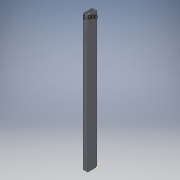
# Autodesk Inventor part: 30in 1x1 Beam
Saved by Autodesk Inventor 2018 (Build 220112000, 112)
## iProperties
Created: 2019-01-16
Part Number: 30in 1x1 Beam
Material: Generic
Document SubType Name: Modeling
Designer: Gabriel
Density: 1 g/cm^3
Appearance: Default
Author: Gabriel
Autodesk Inventor part; units mm, degrees
ref_plane "YZ Plane" through (0, 0, 0) normal (1, 0, 0) x (0, 1, 0)
ref_plane "XZ Plane" through (0, 0, 0) normal (0, 1, 0) x (-1, 0, 0)
ref_plane "XY Plane" through (0, 0, 0) normal (0, 0, 1) x (1, 0, 0)
sketch "Sketch1" plane through (0, 0, 0) normal (0, 1, 0) x (-1, 0, 0)
  line L0 (2.2807, -2.5252) -> (-23.1193, -2.5252)
  line L1 (-23.1193, -2.5252) -> (-23.1193, 48.2748)
  line L2 (-23.1193, 48.2748) -> (2.2807, 48.2748)
  line L3 (2.2807, 48.2748) -> (2.2807, -2.5252)
  line L4 (-19.9443, 0.6498) -> (-0.8943, 0.6498)
  line L5 (-0.8943, 0.6498) -> (-0.8943, 45.0998)
  line L6 (-0.8943, 45.0998) -> (-19.9443, 45.0998)
  line L7 (-19.9443, 45.0998) -> (-19.9443, 0.6498)
  point P0 (0, 0)
  dimension "d0" = 25.4
  dimension "d1" = 50.8
  dimension "d2" = 3.175
  constraints: 16 end point, 4 parallel, 2 perpendicular, 1 horizontal, 3 other
  measures "d0" distance of L1.end L2.end
  measures "d1" distance of L0.end L1.end
  measures "d2" distance between parallel lines of L0 L4
extrude "Extrusion1" add sketch "Sketch1" along normal blind 762
sketch "Sketch3" plane through (-2.2807, 0, 48.2748) normal (0, 0, 1) x (1, 0, 0)
  line L0 (22.225, 0) -> (3.175, 0) construction
  line L1 (12.7, 0) -> (12.7, 12.7) construction
  line L2 (12.7, 12.7) -> (12.7, 38.1) construction
  line L3 (12.7, 38.1) -> (12.7, 63.5) construction
  circle A0 centre (12.7, 63.5) radius 2.5797
  circle A1 centre (12.7, 38.1) radius 2.5797
  circle A2 centre (12.7, 12.7) radius 2.5797
  line L4 (12.7, 685.8) -> (12.7, 673.1) construction
  circle A3 centre (12.7, 673.1) radius 2.5797
  line L5 (12.7, 673.1) -> (12.7, 647.7) construction
  line L6 (12.7, 647.7) -> (12.7, 622.3) construction
  circle A4 centre (12.7, 647.7) radius 2.5797
  circle A5 centre (12.7, 622.3) radius 2.5797
  point P0 (2.2807, 0)
  dimension "d19" = 12.7
  dimension "d20" = 25.4
  dimension "d21" = 25.4
  dimension "d22" = 5.1594
  dimension "d23" = 5.1594
  dimension "d24" = 5.1594
  dimension "d38" = 12.7
  dimension "d39" = 5.1594
  dimension "d40" = 25.4
  dimension "d41" = 25.4
  dimension "d42" = 5.1594
  dimension "d43" = 5.1594
  constraints: 12 end point, 6 centre point, 6 coincident, 3 point on line, 2 vertical, 1 midpoint
  measures "d19" distance of L1.start L1.end
  measures "d20" distance of L1.end L2.end
  measures "d21" distance of L2.end L3.end
  measures "d22" diameter of A0
  measures "d23" diameter of A1
  measures "d24" diameter of A2
  measures "d38" distance of L4.start L4.end
  measures "d39" diameter of A3
  measures "d40" distance of L5.start L5.end
  measures "d41" distance of L5.end L6.end
  measures "d42" diameter of A4
  measures "d43" diameter of A5
extrude "Extrusion3" cut sketch "Sketch3" against normal blind 762
sketch "Sketch4" plane through (23.1193, 0, 48.2748) normal (1, 0, 0) x (0, 0, -1)
  line L0 (3.175, 762) -> (47.625, 762) construction
  line L1 (25.4, 762) -> (25.4, 736.6) construction
  point P0 (48.2748, 0)
  dimension "d44" = 25.4
  constraints: 2 end point, 1 midpoint, 1 vertical
  measures "d44" distance of L1.start L1.end
sketch "Sketch5" plane through (-2.2807, 0, -2.5252) normal (-1, 0, 0) x (0, 0, 1)
  circle A0 centre (25.4, 12.7) radius 2.5797 projected
  line L0 (50.8, 0) -> (50.8, 762) projected
  circle A1 centre (25.4, 38.1) radius 2.5797 construction
  line L1 (50.8, 38.1) -> (38.1, 38.1) construction
  circle A2 centre (25.4, 63.5) radius 2.5797 construction
  line L2 (50.8, 63.5) -> (38.1, 63.5) construction
  circle A3 centre (38.1, 63.5) radius 2.5797
  circle A4 centre (38.1, 38.1) radius 2.5797
  circle A5 centre (38.1, 12.7) radius 2.5797
  line L3 (38.1, 12.7) -> (50.8, 12.7) construction
  circle A6 centre (25.4, 622.3) radius 2.5797 construction
  line L4 (50.8, 622.3) -> (38.1, 622.3) construction
  circle A7 centre (25.4, 647.7) radius 2.5797 construction
  line L5 (50.8, 647.7) -> (38.1, 647.7) construction
  circle A8 centre (25.4, 673.1) radius 2.5797 construction
  line L6 (50.8, 673.1) -> (38.1, 673.1) construction
  circle A9 centre (38.1, 647.7) radius 2.5797
  circle A10 centre (38.1, 622.3) radius 2.5797
  circle A11 centre (38.1, 673.1) radius 2.5797
  point P0 (2.5252, 0)
  dimension "d46" = 12.7
  dimension "d47" = 12.7
  dimension "d48" = 5.1594
  dimension "d49" = 5.1594
  dimension "d50" = 5.1594
  dimension "d51" = 12.7
  dimension "d52" = 12.7
  dimension "d53" = 12.7
  dimension "d54" = 5.1594
  dimension "d55" = 5.1594
  dimension "d56" = 5.1594
  constraints: 12 end point, 6 centre point, 6 point on line, 5 coincident, 1 perpendicular
  measures "d46" distance of L1.start L1.end
  measures "d47" distance of L2.start L2.end
  measures "d48" diameter of A3
  measures "d49" diameter of A4
  measures "d50" diameter of A5
  measures "d51" distance of L4.start L4.end
  measures "d52" distance of L5.start L5.end
  measures "d53" distance of L6.start L6.end
  measures "d54" diameter of A9
  measures "d55" diameter of A10
  measures "d56" diameter of A11
extrude "Extrusion4" cut sketch "Sketch5" against normal blind 762 contours A3 | A4 | A5 | A9 | A10 | A11
sketch "Sketch6" plane through (-2.2807, 0, -2.5252) normal (-1, 0, 0) x (0, 0, 1)
  line L0 (47.625, 762) -> (3.175, 762) construction
  line L1 (25.4, 762) -> (25.4, 736.6) construction
  circle A0 centre (25.4, 736.6) radius 14.2875
  point P0 (2.5252, 0)
  dimension "d59" = 25.4
  dimension "d60" = 28.575
  constraints: 2 end point, 1 centre point, 1 coincident, 1 midpoint, 1 vertical
  measures "d59" distance of L1.start L1.end
  measures "d60" diameter of A0
extrude "Extrusion5" cut sketch "Sketch6" against normal blind 304.8
sketch "Sketch7" plane through (-2.2807, 0, -2.5252) normal (-1, 0, 0) x (0, 0, 1)
  circle A0 centre (38.1, 12.7) radius 2.5797 construction
  line L0 (38.1, 12.7) -> (38.1, 114.3) construction
  line L1 (38.1, 12.7) -> (38.1, 190.5) construction
  line L2 (38.1, 190.5) -> (12.7, 190.5) construction
  line L3 (38.1, 114.3) -> (12.7, 114.3) construction
  circle A1 centre (38.1, 190.5) radius 2.5797
  circle A2 centre (12.7, 190.5) radius 2.5797
  circle A3 centre (38.1, 114.3) radius 2.5797
  circle A4 centre (12.7, 114.3) radius 2.5797
  point P0 (2.5252, 0)
  dimension "d63" = 101.6
  dimension "d64" = 177.8
  dimension "d65" = 25.4
  dimension "d66" = 25.4
  dimension "d67" = 5.1594
  dimension "d68" = 5.1594
  dimension "d69" = 5.1594
  dimension "d70" = 5.1594
  constraints: 8 end point, 4 centre point, 4 coincident, 2 horizontal, 1 point on line, 1 vertical
  measures "d63" distance of L0.start L0.end
  measures "d64" distance of L0.start L1.end
  measures "d65" distance of L1.end L2.end
  measures "d66" distance of L0.end L3.end
  measures "d67" diameter of A1
  measures "d68" diameter of A2
  measures "d69" diameter of A3
  measures "d70" diameter of A4
extrude "Extrusion6" cut sketch "Sketch7" against normal blind 50.8
body "Solid1"
